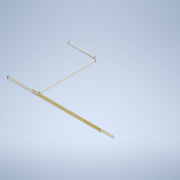
# Autodesk Inventor part: StationDividerBend-ver1-1111-2021
Saved by Autodesk Inventor 2021 (Build 250183000, 183)
## iProperties
Created: 2021-03-02
Part Number: StationDividerBend-ver1-1111-2021
Material: Generic
Document SubType Name: Modeling
Designer: CMurray
Density: 1 g/cm^3
Appearance: Default
Author: CMurray
Autodesk Inventor part; units mm, degrees
ref_plane "YZ Plane" through (0, 0, 0) normal (1, 0, 0) x (0, 1, 0)
ref_plane "XZ Plane" through (0, 0, 0) normal (0, 1, 0) x (-1, 0, 0)
sketch "Sketch1" plane through (0, 0, 0) normal (1, 0, 0) x (0, 1, 0)
  circle A0 centre (0, 0) radius 12.7
  circle A1 centre (0, 0) radius 15.875
  dimension "d0" = 25.4
  dimension "d1" = 3.175
  constraints: 2 centre point, 1 coincident
  measures "d0" diameter of A0
  measures "d1" radial gap between concentric circles of A0 A1
extrude "Extrusion1" add sketch "Sketch1" along normal blind 457.2
ref_plane "Work Plane1" through (0, 0, -15.875) normal (0, 0, 1) x (1, 0, 0)
sketch "Sketch3" plane through (0, 0, -15.875) normal (0, 0, 1) x (1, 0, 0)
  line L0 (127, -49.119) -> (127, 55.4129)
  line L1 (0, -15.875) -> (0, 15.875) projected
  point P0 (0, 0)
  dimension "d7" = 127
  constraints: 2 end point, 1 vertical
  measures "d7" distance between parallel lines of L0 L1
bend part "Bend Part1" radius 25.4 angle 90 line through (127, -49.119, -15.875) along (0, 1, 0) centre toward (0, 0, -1) moving side (1, 0, 0) both sides no
sketch "Sketch4" plane through (168.275, 0, -331.5768) normal (0, 0, -1) x (-1, 0, 0)
  circle A0 centre (0, 0) radius 12.7
  circle A1 centre (0, 0) radius 15.875
  point P0 (168.275, 0)
  dimension "d10" = 3.175
  constraints: 2 centre point
  measures "d10" radial gap between concentric circles of A0 A1
extrude "Extrusion3" add sketch "Sketch4" along normal blind 166.9034
sketch "Sketch5" plane through (0, 0, 0) normal (-1, 0, 0) x (0, 0, 1)
  circle A0 centre (0, 0) radius 12.7
  circle A1 centre (0, 0) radius 15.875
  dimension "d13" = 3.175
  constraints: 2 centre point, 1 coincident
  measures "d13" radial gap between concentric circles of A0 A1
extrude "Extrusion4" add sketch "Sketch5" along normal blind 1016
ref_plane "Work Plane2" through (0, 0, -15.875) normal (0, 0, 1) x (1, 0, 0)
sketch "Sketch6" plane through (0, 0, -15.875) normal (0, 0, 1) x (1, 0, 0)
  line L0 (-889, -31.575) -> (-889, 43.9679)
  line L1 (-1016, 15.875) -> (-1016, -15.875) projected
  point P0 (0, 0)
  dimension "d16" = 127
  constraints: 2 end point, 1 vertical
  measures "d16" distance between parallel lines of L0 L1
bend part "Bend Part2" radius 25.4 angle 90 line through (-889, -31.575, -15.875) along (0, 1, 0) centre toward (0, 0, -1) moving side (1, 0, 0) both sides no
sketch "Sketch7" plane through (-1016, 0, 0) normal (-1, 0, 0) x (0, 0, 1)
  circle A0 centre (0, 0) radius 12.7
  circle A1 centre (0, 0) radius 15.875
  dimension "d19" = 3.175
  constraints: 2 centre point, 1 coincident
  measures "d19" radial gap between concentric circles of A0 A1
extrude "Extrusion5" add sketch "Sketch7" along normal blind 330.2
body "Solid1"
